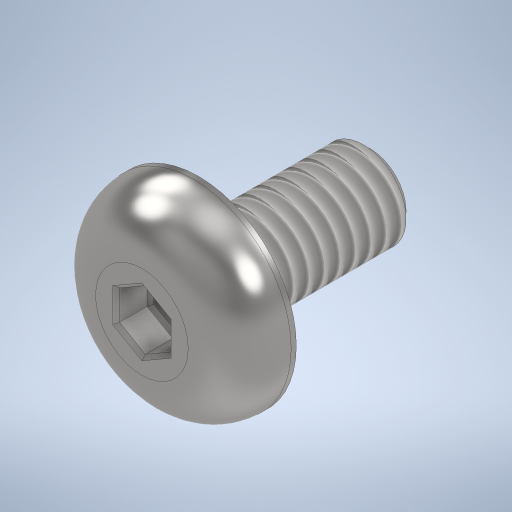
# Autodesk Inventor part: rapoukHexagonScrewM2,5v0
Saved by Autodesk Inventor 2024 (Build 280153000, 153)
## iProperties
Created: 2024-01-30
Part Number: rapoukHexagonScrewM2,5v0
Material: Steel, Carbon
Document SubType Name: Modeling
Designer: Roman Suk
Density: 7.85 g/cm^3
Appearance: Semi-Polished
MASSSFP: 400 g
SFP: 4HR
Author: Roman Suk
Autodesk Inventor part; units mm, degrees
ref_plane "YZ Plane" through (0, 0, 0) normal (1, 0, 0) x (0, 1, 0)
ref_plane "XZ Plane" through (0, 0, 0) normal (0, 1, 0) x (-1, 0, 0)
ref_plane "XY Plane" through (0, 0, 0) normal (0, 0, 1) x (1, 0, 0)
sketch "Sketch2" plane through (0, 0, 0) normal (0, 1, 0) x (-1, 0, 0)
  line L0 (0, 0) -> (2.85, 0)
  line L1 (2.85, 0) -> (2.85, -1.65)
  line L2 (2.85, -1.65) -> (1.25, -1.65)
  line L3 (1.25, -1.65) -> (1.25, -6.65)
  line L4 (1.25, -6.65) -> (0, -6.65)
  line L5 (0, 0) -> (0, -6.65)
  dimension "d9" = 2.85
  dimension "d10" = 1.65
  dimension "d12" = 5
  dimension "d19" = 2.5
  constraints: 12 end point, 3 perpendicular, 2 horizontal, 1 vertical
  measures "d9" distance of L0.start L0.end
  measures "d10" distance of L0.end L1.end
  measures "d12" distance of L2.end L3.end
  measures "d19" diameter of L3 L5
revolve "Revolution1" add sketch "Sketch2" angle 360 about axis through (0, 0, 0) along (0, 0, -1)
fillet "Fillet1" radius 1.5 1 edges at (2.85, 0, 0)
chamfer "Chamfer1" distance 0.2 angle 45 1 edges at (1.25, 0, -6.65)
thread "Thread1" size "M2.5x0.45" class "6g" standard "ANSI Metric M Profile" full length
sketch "Sketch4" plane through (0, 0, 0) normal (0, 0, 1) x (1, 0, 0)
  line L0 (0, 0.866) -> (0.75, 0.433)
  line L1 (0.75, 0.433) -> (0.75, -0.433)
  line L2 (0.75, -0.433) -> (0, -0.866)
  line L3 (0, -0.866) -> (-0.75, -0.433)
  line L4 (-0.75, -0.433) -> (-0.75, 0.433)
  line L5 (-0.75, 0.433) -> (0, 0.866)
  circle A0 centre (0, 0) radius 1.05 projected
  point P0 (0, 0)
  dimension "d22" = 1.5
  dimension "d30" = 0.433
  constraints: 12 end point, 1 coincident, 13 other
  measures "d22" distance between parallel lines of L1 L4
  measures "d30" vertical distance of A0.centre L1.end
extrude "Extrusion2" cut sketch "Sketch4" against normal blind 1 contours L0 L1 L2 L3 L4 L5
chamfer "Chamfer2" distance 0.1 angle 45 12 edges at (-0.75, 0, 0) (-0.375, 0.6495, 0) (0.375, 0.6495, 0) (0.75, 0, 0) (0.375, -0.6495, 0) (-0.375, -0.6495, 0) (-0.375, 0.6495, -1) (-0.75, 0, -1) (-0.375, -0.6495, -1) (0.375, -0.6495, -1) (0.75, 0, -1) (0.375, 0.6495, -1)
body "Solid2"
